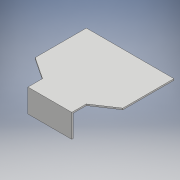
# Autodesk Inventor part: Body Back
Saved by Autodesk Inventor 2018 (Build 220112000, 112)
## iProperties
Created: 2018-04-26
Part Number: Body Back
Material: Generic
Document SubType Name: Modeling
Designer: HP
Density: 1 g/cm^3
Appearance: Default
Author: HP
Autodesk Inventor part; units mm, degrees
ref_plane "YZ Plane" through (0, 0, 0) normal (1, 0, 0) x (0, 1, 0)
ref_plane "XZ Plane" through (0, 0, 0) normal (0, 1, 0) x (-1, 0, 0)
ref_plane "XY Plane" through (0, 0, 0) normal (0, 0, 1) x (1, 0, 0)
sketch "Sketch1" plane through (0, 0, 0) normal (0, 0, 1) x (1, 0, 0)
  line L0 (60, 40) -> (60, 110)
  line L1 (60, 110) -> (-60, 110)
  line L2 (-60, 110) -> (-60, 40)
  line L3 (-30, 0) -> (30, 0)
  line L4 (30, 0) -> (30, 20)
  line L5 (-30, 20) -> (-30, 0)
  line L6 (-60, 40) -> (-30, 20)
  line L7 (30, 20) -> (60, 40)
  point P0 (0, 0)
  dimension "d4" = 120
  dimension "d5" = 70
  dimension "d7" = 20
  dimension "d8" = 60
  constraints: 16 end point, 2 parallel, 1 horizontal, 1 perpendicular
  measures "d4" distance of L1.end L0.end
  measures "d5" distance of L0.end L0.start
  measures "d7" distance of L4.end L3.end
  measures "d8" distance between parallel lines of L4 L5
extrude "Extrusion1" add sketch "Sketch1" along normal blind 2
sketch "Sketch2" plane through (-30, 0, 0) normal (0, -1, 0) x (1, 0, 0)
  line L0 (60, 0) -> (60, 2) projected
  line L1 (60, 0) -> (0, 0)
  line L2 (0, 0) -> (0, -30)
  line L3 (0, -30) -> (60, -30)
  line L4 (60, -30) -> (60, 0)
  dimension "d11" = 60
  dimension "d12" = 30
  constraints: 8 end point, 2 parallel, 1 horizontal, 1 perpendicular
  measures "d11" distance of L3.end L2.end
  measures "d12" distance of L2.end L1.end
extrude "Extrusion2" add sketch "Sketch2" against normal blind 2
body "Solid1"
